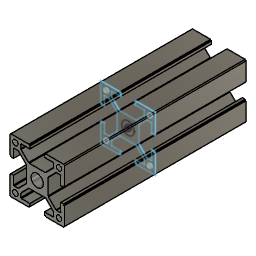
Aluminium extrusion 3030 v2 (Autodesk Fusion 360 design; units mm, degrees)
Autodesk Fusion 360 part; units mm, degrees
sketch "Sketch1" plane through (0, 0, 0) normal (0, 1, 0) x (1, 0, 0)
  circle A0 centre (0, 0) radius 3.4
  line L0 (15, -15) -> (4.5, -15)
  line L1 (4.5, -15) -> (4.5, -14.5)
  line L2 (4.5, -14.5) -> (4, -14.5)
  line L3 (4, -14.5) -> (4, -13)
  line L4 (4, -13) -> (9, -13)
  line L5 (15, -15) -> (15, -4.5)
  line L6 (15, -4.5) -> (14.5, -4.5)
  line L7 (14.5, -4.5) -> (14.5, -4)
  line L8 (14.5, -4) -> (13, -4)
  line L9 (13, -4) -> (13, -9)
  line L10 (13, -9) -> (10.4142, -9)
  line L11 (9, -13) -> (9, -10.4142)
  line L12 (9, -10.4142) -> (4.5858, -6)
  line L13 (10.4142, -9) -> (6, -4.5858)
  line L14 (13, 4) -> (13, 9)
  line L15 (14.5, 4) -> (13, 4)
  line L16 (9, 10.4142) -> (4.5858, 6)
  line L17 (15, 4.5) -> (14.5, 4.5)
  line L18 (4.5, 15) -> (4.5, 14.5)
  line L19 (4, 14.5) -> (4, 13)
  line L20 (10.4142, 9) -> (6, 4.5858)
  line L21 (13, 9) -> (10.4142, 9)
  line L22 (15, 15) -> (4.5, 15)
  line L23 (4, 13) -> (9, 13)
  line L24 (4.5, 14.5) -> (4, 14.5)
  line L25 (15, 15) -> (15, 4.5)
  line L26 (14.5, 4.5) -> (14.5, 4)
  line L27 (9, 13) -> (9, 10.4142)
  line L28 (-4, 13) -> (-9, 13)
  line L29 (-4, 14.5) -> (-4, 13)
  line L30 (-10.4142, 9) -> (-6, 4.5858)
  line L31 (-4.5, 15) -> (-4.5, 14.5)
  line L32 (-15, 4.5) -> (-14.5, 4.5)
  line L33 (-14.5, 4) -> (-13, 4)
  line L34 (-9, 10.4142) -> (-4.5858, 6)
  line L35 (-9, 13) -> (-9, 10.4142)
  line L36 (-15, 15) -> (-15, 4.5)
  line L37 (-13, 4) -> (-13, 9)
  line L38 (-14.5, 4.5) -> (-14.5, 4)
  line L39 (-15, 15) -> (-4.5, 15)
  line L40 (-4.5, 14.5) -> (-4, 14.5)
  line L41 (-13, 9) -> (-10.4142, 9)
  line L42 (-13, -4) -> (-13, -9)
  line L43 (-14.5, -4) -> (-13, -4)
  line L44 (-9, -10.4142) -> (-4.5858, -6)
  line L45 (-15, -4.5) -> (-14.5, -4.5)
  line L46 (-4.5, -15) -> (-4.5, -14.5)
  line L47 (-4, -14.5) -> (-4, -13)
  line L48 (-10.4142, -9) -> (-6, -4.5858)
  line L49 (-13, -9) -> (-10.4142, -9)
  line L50 (-15, -15) -> (-4.5, -15)
  line L51 (-4, -13) -> (-9, -13)
  line L52 (-4.5, -14.5) -> (-4, -14.5)
  line L53 (-15, -15) -> (-15, -4.5)
  line L54 (-14.5, -4.5) -> (-14.5, -4)
  line L55 (-9, -13) -> (-9, -10.4142)
  line L56 (4.5858, -6) -> (-4.5858, -6)
  line L57 (-6, -4.5858) -> (-6, 4.5858)
  line L58 (-4.5858, 6) -> (4.5858, 6)
  line L59 (6, 4.5858) -> (6, -4.5858)
  circle A1 centre (12, -12) radius 1.5
  circle A2 centre (12, 12) radius 1.5
  circle A3 centre (-12, 12) radius 1.5
  circle A4 centre (-12, -12) radius 1.5
  dimension "d1" = 6.8
  dimension "d7" = 360
  dimension "d8" = 3
  dimension "d9" = 8
  dimension "d10" = 30
  dimension "d11" = 12
  dimension "d22" = 18
  dimension "d23" = 2
  dimension "d24" = 7
  constraint coincident A0.centre origin
  constraint perpendicular L0 L1
  constraint perpendicular L0 L3
  constraint perpendicular L3 L4
  constraint perpendicular L0 L5
  constraint perpendicular L5 L6
  constraint perpendicular L0 L7
  constraint perpendicular L7 L8
  constraint perpendicular L8 L9
  constraint perpendicular L9 L10
  constraint perpendicular L4 L11
  measures "d1" diameter of A0
  measures "d8" diameter of A1
  measures "d9" distance of L8 L15
  measures "d10" distance of L0 L22
  measures "d11" distance of L57 L59
  measures "d22" distance of L11 L55
  measures "d23" distance of L5 L9
  measures "d24" distance of L4 L56
extrude "Extrude1" add sketch "Sketch1" along normal mid plane 100
fillet "Fillet1" radius 0.5 4 edges at (-15, 0, 15) (15, 0, 15) (-15, 0, -15) (15, 0, -15)
fillet "Fillet2" radius 0.3 8 edges at (-13, 0, -9) (-9, 0, -13) (9, 0, -13) (13, 0, -9) (13, 0, 9) (9, 0, 13) (-9, 0, 13) (-13, 0, 9)
fillet "Fillet3" radius 0.3 8 edges at (-10.4142, 0, -9) (-9, 0, -10.4142) (9, 0, -10.4142) (10.4142, 0, -9) (-9, 0, 10.4142) (-10.4142, 0, 9) (9, 0, 10.4142) (10.4142, 0, 9)
fillet "Fillet4" radius 0.5 8 edges at (-4.5858, 0, 6) (6, 0, 4.5858) (6, 0, -4.5858) (4.5858, 0, 6) (-6, 0, 4.5858) (-6, 0, -4.5858) (4.5858, 0, -6) (-4.5858, 0, -6)
